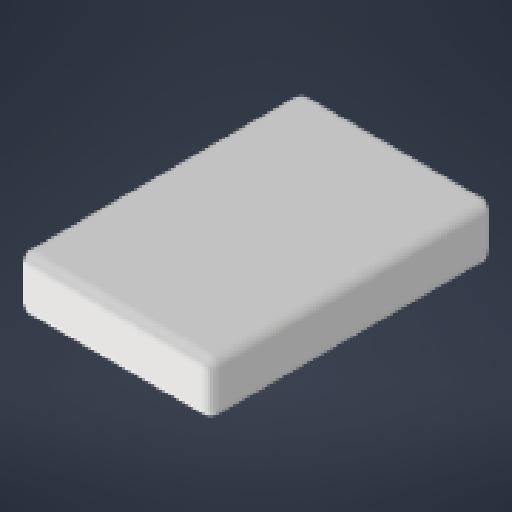
# Autodesk Inventor part: ColdBye_Battery
Saved by Autodesk Inventor 2026.2 (Build 302298000, 298)
## iProperties
Created: 2026-03-01
Part Number: ColdBye_Battery
Material: Generic
Document SubType Name: Modeling
Designer: vckot
Density: 1 g/cm^3
Appearance: Default
Author: vckot
Autodesk Inventor part; units mm, degrees
ref_plane "YZ Plane" through (0, 0, 0) normal (1, 0, 0) x (0, 1, 0)
ref_plane "XZ Plane" through (0, 0, 0) normal (0, 1, 0) x (-1, 0, 0)
ref_plane "XY Plane" through (0, 0, 0) normal (0, 0, 1) x (1, 0, 0)
sketch "Sketch1" plane through (0, 0, 0) normal (0, 1, 0) x (-1, 0, 0)
  line L0 (-32.004, 46.99) -> (32.004, 46.99)
  line L1 (32.004, 46.99) -> (32.004, -46.99)
  line L2 (32.004, -46.99) -> (-32.004, -46.99)
  line L3 (-32.004, -46.99) -> (-32.004, 46.99)
  line L4 (-32.004, 46.99) -> (32.004, -46.99) construction
  line L5 (32.004, 46.99) -> (-32.004, -46.99) construction
  point P0 (0, 0)
  dimension "d0" = 64.008
  dimension "d1" = 93.98
  constraints: 12 end point, 2 midpoint, 2 parallel, 1 horizontal, 1 perpendicular
  measures "d0" distance of L1.end L2.end
  measures "d1" distance of L0.end L1.end
extrude "Extrusion1" add sketch "Sketch1" along normal mid plane 18.034
fillet "Fillet1" radius 3.175 12 edges at (32.004, 9.017, 0) (32.004, -9.017, 0) (32.004, 0, 46.99) (-32.004, 9.017, 0) (0, 9.017, 46.99) (-32.004, 0, 46.99) (0, -9.017, 46.99) (-32.004, -9.017, 0) (-32.004, 0, -46.99) (0, 9.017, -46.99) (0, -9.017, -46.99) (32.004, 0, -46.99)
body "Solid1"
